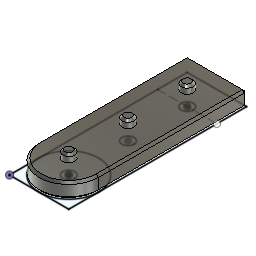
Chop Saw Guide (Autodesk Fusion 360 design; units mm, degrees)
Autodesk Fusion 360 part; units mm, degrees
sketch "Sketch1" plane through (0, 0, 0) normal (0, 0, 1) x (1, 0, 0)
  line L0 (0, 0) -> (25.4, 0)
  line L1 (25.4, 0) -> (25.4, 63.5)
  line L2 (25.4, 63.5) -> (0, 63.5) construction
  line L3 (0, 63.5) -> (0, 0)
  line L4 (25.4, 63.5) -> (25.4, 76.2)
  line L5 (25.4, 76.2) -> (0, 76.2)
  line L6 (0, 76.2) -> (0, 63.5)
  circle A0 centre (12.7, 63.5) radius 2.54
  circle A1 centre (12.7, 38.1) radius 2.54
  circle A2 centre (12.7, 12.7) radius 2.54
  circle A3 centre (12.7, 12.7) radius 12.7
  dimension "d8" = 25.4
  dimension "d9" = 63.5
  dimension "d11" = 12.7
  dimension "d12" = 5.08
  dimension "d15" = 25.4
  dimension "d16" = 0
  constraint horizontal L0
  constraint vertical L1
  constraint horizontal L2
  constraint vertical L3
  constraint coincident L0.start L3.end
  constraint vertical L4
  constraint horizontal L5
  constraint vertical L6
  constraint collinear L1 L4
  constraint midpoint L2 A0.centre
  constraint concentric A2 A3
  constraint tangent L3 A3
  measures "d8" distance of L0.start L0.end
  measures "d9" distance of L0.start L2.end
  measures "d11" distance of L2.end L5.end
  measures "d12" diameter of A0
extrude "Extrude1" add sketch "Sketch1" along normal blind 6.35 contours A3 | L1 L3 L4 L5 L6 A3 | A0 | A1 | A2
extrude "Extrude2" add sketch "Sketch1" along normal blind 3.175 from surface at 6.35 contours A0 | A1 | A2
chamfer "Chamfer1" distance 0.9 angle 45 9 edges at (10.3319, 11.7815, 9.525) (10.3319, 37.1815, 9.525) (10.3319, 62.5815, 9.525) (25.4, 76.2, 3.175) (0, 76.2, 3.175) (12.7, 76.2, 6.35) (0, 44.45, 6.35) (12.7, 0, 6.35) (25.4, 44.45, 6.35) 1 faces at (8.4667, 33.8667, 0)
equation "CUT_DISTANCE = 0.5 in" comment "Cutting edge tip"
equation "TUBE_WIDTH = 1 in" comment "Width of  tubing"
equation "PIN_SPACING = 1 in" comment "Spacing of holes"
equation "PIN_DIAMETER = 0.2 in" comment "Pin size"
equation "GUIDE_THICKNESS = 0.25 in" comment "Thickness of guide"
equation "PIN_LENGTH = 0.125 in" comment "Height of pin"
equation "PRINTER_LAYER_HEIGHT = 0.3 mm" comment "Layer height for chamfer"
equation "d8 = TUBE_WIDTH"
equation "d9 = PIN_SPACING * ( PIN_COUNT - 0.5 )"
equation "PIN_COUNT = 3" comment "# of pins"
equation "d11 = CUT_DISTANCE"
equation "d12 = PIN_DIAMETER"
equation "d13 = PIN_COUNT"
equation "d15 = PIN_SPACING"
equation "d17 = GUIDE_THICKNESS"
equation "d20 = PIN_LENGTH"
equation "d22 = PRINTER_LAYER_HEIGHT * 3"
